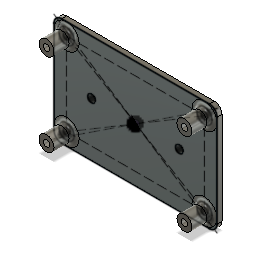
VPForce_Board_Holder (Autodesk Fusion 360 design; units mm, degrees)
Autodesk Fusion 360 part; units mm, degrees
sketch "Sketch1" plane through (0, 0, 0) normal (0, 0, 1) x (1, 0, 0)
  line L0 (27.5, 16.5) -> (-27.5, 16.5) construction
  line L1 (-27.5, 16.5) -> (-27.5, -16.5) construction
  line L2 (-27.5, -16.5) -> (27.5, -16.5) construction
  line L3 (27.5, -16.5) -> (27.5, 16.5) construction
  line L4 (27.5, 16.5) -> (-27.5, -16.5) construction
  line L5 (-27.5, 16.5) -> (27.5, -16.5) construction
  line L6 (-29.5, 21.5) -> (29.5, 21.5)
  line L7 (32.5, 18.5) -> (32.5, -18.5)
  line L8 (29.5, -21.5) -> (-29.5, -21.5)
  line L9 (-32.5, -18.5) -> (-32.5, 18.5)
  line L10 (-32.5, 21.5) -> (32.5, -21.5) construction
  line L11 (32.5, 21.5) -> (-32.5, -21.5) construction
  arc A0 (-29.5, 21.5) -> (-32.5, 18.5) centre (-29.5, 18.5) ccw
  arc A1 (-32.5, -18.5) -> (-29.5, -21.5) centre (-29.5, -18.5) ccw
  arc A2 (29.5, -21.5) -> (32.5, -18.5) centre (29.5, -18.5) ccw
  arc A3 (32.5, 18.5) -> (29.5, 21.5) centre (29.5, 18.5) ccw
  circle A4 centre (27.5, -16.5) radius 3
  circle A5 centre (27.5, -16.5) radius 1.264
  circle A6 centre (27.5, 16.5) radius 3
  circle A7 centre (27.5, 16.5) radius 1.264
  circle A8 centre (-27.5, -16.5) radius 3
  circle A9 centre (-27.5, -16.5) radius 1.264
  circle A10 centre (-27.5, 16.5) radius 3
  circle A11 centre (-27.5, 16.5) radius 1.264
  circle A12 centre (17.5, 0) radius 1.5
  circle A13 centre (-17.5, 0) radius 1.5
  dimension "d1" = 55
  dimension "d2" = 33
  dimension "d3" = 65
  dimension "d4" = 43
  dimension "d5" = 3
  dimension "d6" = 6
  dimension "d7" = 2.528
  dimension "d8" = 6
  dimension "d9" = 2.528
  dimension "d10" = 2.528
  dimension "d11" = 6
  dimension "d12" = 2.528
  dimension "d13" = 6
  dimension "d14" = 17.5
  dimension "d15" = 3
  dimension "d16" = 17.5
  dimension "d17" = 3
  constraint horizontal L0
  constraint perpendicular L0 L1
  constraint parallel L0 L2
  constraint parallel L1 L3
  constraint coincident L4 origin
  constraint coincident L5 origin
  constraint horizontal L6
  constraint perpendicular L6 L7
  constraint parallel L6 L8
  constraint parallel L7 L9
  constraint coincident L10 origin
  constraint coincident L11 origin
  constraint coincident L10.start L6
  constraint coincident L10.start L9
  constraint tangent L6 A0
  constraint tangent L9 A0
  constraint coincident L11.end L9
  constraint coincident L11.end L8
  constraint tangent L9 A1
  constraint tangent L8 A1
  constraint equal A0 A1
  constraint coincident L10.end L8
  constraint coincident L10.end L7
  constraint tangent L8 A2
  constraint tangent L7 A2
  constraint equal A0 A2
  constraint coincident L11.start L7
  constraint coincident L11.start L6
  constraint tangent L7 A3
  constraint tangent L6 A3
  constraint equal A0 A3
  constraint coincident L2.end L3.start
  constraint concentric A4 A5
  constraint coincident L0.start L3.end
  constraint concentric A6 A7
  constraint coincident L1.end L2.start
  constraint concentric A8 A9
  constraint coincident L0.end L1.start
  constraint concentric A10 A11
  constraint horizontal origin A12.centre
  constraint horizontal origin A13.centre
  measures "d1" distance of L1.end L2.end
  measures "d2" distance of L0.end L1.end
  measures "d3" distance of L10.end L11.end
  measures "d4" distance of L11.start L10.end
  measures "d5" radius of A0
  measures "d6" diameter of A4
  measures "d7" diameter of A5
  measures "d8" diameter of A6
  measures "d9" diameter of A7
  measures "d10" diameter of A9
  measures "d11" diameter of A8
  measures "d12" diameter of A11
  measures "d13" diameter of A10
  measures "d14" distance of origin A12.centre
  measures "d15" diameter of A12
  measures "d16" distance of origin A13.centre
  measures "d17" diameter of A13
extrude "Extrude1" add sketch "Sketch1" against normal blind 2 contours L6 L7 L8 L9 A0 A1 A2 A3 | A4 | A5 | A6 | A7 | A8 | A9 | A10 | A11
extrude "Extrude2" add sketch "Sketch1" along normal blind 8 contours A4 | A6 | A8 | A10
fillet "Fillet1" radius 2 4 edges at (-30.297, 17.5848, 0) (-30.297, -15.4152, 0) (24.703, -15.4152, 0) (24.703, 17.5848, 0)
equation "d7 = ( 1.264 * 2 ) * 1 mm"
equation "d8 = d6"
equation "d9 = d7"
equation "d10 = d7"
equation "d11 = d6"
equation "d12 = d7"
equation "d13 = d6"
equation "d14 = ( 35 / 2 ) * 1 mm"
equation "d16 = d14"
equation "d17 = d15"
